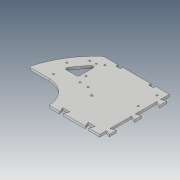
# Autodesk Inventor part: FR_bottomPlate
Saved by Autodesk Inventor 2018 (Build 220112000, 112)
## iProperties
Created: 2020-01-08
Part Number: FR_bottomPlate
Material: Generic
Document SubType Name: Modeling
Designer: anirudh
Density: 1 g/cm^3
Appearance: Default
Author: anirudh
Autodesk Inventor part; units mm, degrees
ref_plane "YZ Plane" through (0, 0, 0) normal (1, 0, 0) x (0, 1, 0)
ref_plane "XZ Plane" through (0, 0, 0) normal (0, 1, 0) x (-1, 0, 0)
ref_plane "XY Plane" through (0, 0, 0) normal (0, 0, 1) x (1, 0, 0)
sketch "Sketch1" plane through (0, 0, 0) normal (0, 1, 0) x (-1, 0, 0)
  arc A0 (-134.4042, 152.4) -> (-189.4285, 73.533) centre (0, 0) ccw
  arc A1 (-189.4285, -73.533) -> (-134.4042, -152.4) centre (0, 0) ccw
  arc A2 (-134.4042, 152.4) -> (-189.4285, 73.533) centre (0, 0) ccw
  arc A3 (-189.4285, -73.533) -> (-134.4042, -152.4) centre (0, 0) ccw
  arc A4 (214.8285, 73.533) -> (159.8042, 152.4) centre (25.4, 0) ccw
  arc A5 (159.8042, -152.4) -> (214.8285, -73.533) centre (25.4, 0) ccw
  arc A6 (214.8285, 73.533) -> (159.8042, 152.4) centre (25.4, 0) ccw
  arc A7 (159.8042, -152.4) -> (214.8285, -73.533) centre (25.4, 0) ccw
  arc A8 (-152.4, -50.8) -> (-152.4, 50.8) centre (-152.4, 0) ccw
  arc A9 (177.8, 50.8) -> (177.8, -50.8) centre (177.8, 0) ccw
  line L0 (177.8, 50.8) -> (222.1476, 50.8)
  line L1 (177.8, -50.8) -> (222.1476, -50.8)
  line L2 (-152.4, 50.8) -> (-196.7476, 50.8)
  line L3 (-152.4, -50.8) -> (-196.7476, -50.8)
  arc A10 (-134.4042, 152.4) -> (-196.7476, 50.8) centre (0, 0) ccw
  arc A11 (-196.7476, -50.8) -> (-134.4042, -152.4) centre (0, 0) ccw
  arc A12 (159.8042, -152.4) -> (222.1476, -50.8) centre (25.4, 0) ccw
  arc A13 (222.1476, 50.8) -> (159.8042, 152.4) centre (25.4, 0) ccw
  circle A14 centre (98.425, -65.0875) radius 2.1
  circle A15 centre (98.425, 65.0875) radius 2.1
  circle A16 centre (-73.025, 65.0875) radius 2.1
  circle A17 centre (-73.025, -65.0875) radius 2.1
  line L4 (-20.32, 152.4) -> (-20.32, 147.32)
  line L5 (-20.32, 147.32) -> (-30.48, 147.32)
  line L6 (-30.48, 147.32) -> (-30.48, 152.4)
  line L7 (-92.5481, 152.4) -> (-92.5481, 147.32)
  line L8 (-92.5481, 147.32) -> (-102.7081, 147.32)
  line L9 (-102.7081, 147.32) -> (-102.7081, 152.4)
  line L10 (-102.7081, 152.4) -> (-134.4042, 152.4)
  line L11 (-60.8521, 152.4) -> (-92.5481, 152.4)
  line L12 (-102.7081, 152.4) -> (-134.4042, 152.4)
  line L13 (-134.4042, 152.4) -> (-102.7081, 152.4)
  line L14 (12.7, 152.4) -> (-20.32, 152.4)
  line L15 (-30.48, 152.4) -> (-60.8521, 152.4)
  line L16 (12.7, 152.4) -> (-20.32, 152.4)
  line L17 (-30.48, 152.4) -> (-92.5481, 152.4)
  line L18 (-92.5481, 152.4) -> (-30.48, 152.4)
  line L19 (-20.32, 152.4) -> (12.7, 152.4)
  line L20 (45.72, 152.4) -> (45.72, 147.32)
  line L21 (45.72, 147.32) -> (55.88, 147.32)
  line L22 (55.88, 147.32) -> (55.88, 152.4)
  line L23 (117.9481, 152.4) -> (117.9481, 147.32)
  line L24 (117.9481, 147.32) -> (128.1081, 147.32)
  line L25 (128.1081, 147.32) -> (128.1081, 152.4)
  line L26 (-20.32, -152.4) -> (-20.32, -147.32)
  line L27 (-20.32, -147.32) -> (-30.48, -147.32)
  line L28 (-30.48, -147.32) -> (-30.48, -152.4)
  line L29 (-92.5481, -152.4) -> (-92.5481, -147.32)
  line L30 (-92.5481, -147.32) -> (-102.7081, -147.32)
  line L31 (-102.7081, -147.32) -> (-102.7081, -152.4)
  line L32 (55.88, -147.32) -> (55.88, -152.4)
  line L33 (45.72, -147.32) -> (55.88, -147.32)
  line L34 (45.72, -152.4) -> (45.72, -147.32)
  line L35 (117.9481, -147.32) -> (128.1081, -147.32)
  line L36 (128.1081, -147.32) -> (128.1081, -152.4)
  line L37 (117.9481, -152.4) -> (117.9481, -147.32)
  line L38 (128.1081, 152.4) -> (159.8042, 152.4)
  line L39 (12.7, 152.4) -> (45.72, 152.4)
  line L40 (55.88, 152.4) -> (117.9481, 152.4)
  line L41 (-102.7081, -152.4) -> (-134.4042, -152.4)
  line L42 (12.7, -152.4) -> (-20.32, -152.4)
  line L43 (-30.48, -152.4) -> (-92.5481, -152.4)
  line L44 (12.7, -152.4) -> (45.72, -152.4)
  line L45 (55.88, -152.4) -> (117.9481, -152.4)
  line L46 (128.1081, -152.4) -> (159.8042, -152.4)
  point P0 (-25.4, -152.4)
  point P1 (50.8, 152.4)
  point P2 (50.8, -152.4)
  point P3 (50.8, -152.4)
  dimension "d22" = 101.6
  dimension "d31" = 4.2
  dimension "d32" = 4.2
  dimension "d34" = 4.2
  constraints: 94 end point, 28 point on circle, 18 centre point, 15 collinear, 12 point on line, 7 perpendicular, 4 coincident, 2 tangent, 1 vertical
  measures "d22" diameter of A9
  measures "d31" diameter of A14
  measures "d32" diameter of A15
  measures "d34" diameter of A17
extrude "Extrusion2" add sketch "Sketch1" along normal blind 5.08
sketch "Sketch2" plane through (0, 5.08, 0) normal (0, 1, 0) x (1, 0, 0)
  arc A0 (-177.8, -50.8) -> (-177.8, 50.8) centre (-177.8, 0) ccw projected
  arc A1 (152.4, 50.8) -> (152.4, -50.8) centre (152.4, 0) ccw projected
  line L0 (-177.8, 0) -> (152.4, 0)
  line L1 (-12.7, 0) -> (-12.7, -152.4)
  line L2 (-12.7, 0) -> (-12.7, 152.4)
  line L3 (20.32, 152.4) -> (-45.72, 152.4) projected
  point P0 (0, 0)
  constraints: 6 end point, 2 midpoint, 1 horizontal
sketch "Sketch4" plane through (0, 5.08, 0) normal (0, 1, 0) x (1, 0, 0)
  circle A0 centre (-12.7, 0) radius 300
  point P0 (-177.8, 0)
  point P1 (152.4, 0)
  constraints: 1 centre point
sketch "Sketch5" plane through (0, 5.08, 0) normal (0, 1, 0) x (1, 0, 0)
  line L0 (101.6, 0) -> (80.9498, 0)
  arc A0 (-177.8, -50.8) -> (-177.8, 50.8) centre (-177.8, 0) ccw projected
  line L1 (-106.3498, 0) -> (-106.3498, -74.5998)
  line L2 (30.48, -152.4) -> (92.5481, -152.4) projected
  line L3 (80.9498, -74.5998) -> (-106.3498, -74.5998)
  line L4 (-55.88, 152.4) -> (-117.9481, 152.4) projected
  line L5 (-106.3498, 74.5998) -> (80.9498, 74.5998)
  circle A1 centre (9.525, -102.362) radius 1.75 projected
  line L6 (20.32, 152.4) -> (-45.72, 152.4) projected
  circle A2 centre (-34.925, -140.4366) radius 1.75 projected
  line L7 (-41.3004, -140.4366) -> (-41.3004, -152.4)
  line L8 (-45.72, -152.4) -> (20.32, -152.4) projected
  circle A3 centre (-34.925, -102.362) radius 1.75 projected
  line L9 (-34.925, -89.6366) -> (-41.3004, -89.6366)
  line L10 (-41.3004, -89.6366) -> (15.9004, -89.6366)
  circle A4 centre (-34.925, 102.362) radius 1.75 projected
  line L11 (-34.925, 89.6366) -> (-41.3004, 89.6366)
  line L12 (-41.3004, 89.6366) -> (15.9004, 89.6366)
  line L13 (-41.3004, -152.4) -> (-41.3004, -89.6366)
  line L14 (-41.3004, 89.6366) -> (-41.3004, 152.4)
  line L15 (15.9004, -152.4) -> (15.9004, -89.6366)
  line L16 (15.9004, 89.6366) -> (15.9004, 152.4)
  line L17 (80.9498, -74.5998) -> (80.9498, 74.5998)
  line L18 (80.9498, 0) -> (80.9498, -74.5998)
  line L19 (-106.3498, -74.5998) -> (-106.3498, 74.5998)
  arc A5 (134.4042, -152.4) -> (196.7476, -50.8) centre (0, 0) ccw projected
  line L20 (102.7081, -152.4) -> (134.4042, -152.4) projected
  line L21 (80.9498, -74.5998) -> (80.9498, -68.2498)
  line L22 (84.1248, -68.2498) -> (119.6848, -68.2498)
  line L23 (119.6848, -68.2498) -> (119.6848, -86.0298)
  line L24 (119.6848, -86.0298) -> (84.1248, -86.0298)
  line L25 (84.1248, -86.0298) -> (84.1248, -68.2498)
  line L26 (152.4, 0) -> (-177.8, 0)
  line L27 (-12.7, 0) -> (-12.7, 50.8)
  line L28 (-109.5248, -68.2498) -> (-145.0848, -68.2498)
  line L29 (-145.0848, -68.2498) -> (-145.0848, -86.0298)
  line L30 (-145.0848, -86.0298) -> (-109.5248, -86.0298)
  line L31 (-109.5248, -86.0298) -> (-109.5248, -68.2498)
  line L32 (84.1248, 68.2498) -> (119.6848, 68.2498)
  line L33 (119.6848, 68.2498) -> (119.6848, 86.0298)
  line L34 (119.6848, 86.0298) -> (84.1248, 86.0298)
  line L35 (84.1248, 86.0298) -> (84.1248, 68.2498)
  line L36 (-109.5248, 86.0298) -> (-109.5248, 68.2498)
  line L37 (-145.0848, 86.0298) -> (-109.5248, 86.0298)
  line L38 (-145.0848, 68.2498) -> (-145.0848, 86.0298)
  line L39 (-109.5248, 68.2498) -> (-145.0848, 68.2498)
  line L40 (15.9004, -152.4) -> (15.9004, -133.35)
  line L41 (80.9498, -74.5998) -> (63.1698, -74.5998)
  line L42 (63.1698, -82.1182) -> (63.1698, -133.35)
  line L43 (63.1698, -133.35) -> (15.9004, -133.35)
  line L44 (0, -82.1182) -> (63.1698, -82.1182)
  line L45 (84.1248, -133.35) -> (117.6036, -133.35)
  line L46 (84.1248, -133.35) -> (84.1248, -86.0298)
  line L47 (84.1248, -86.0298) -> (155.6011, -86.0298)
  arc A6 (134.4042, -152.4) -> (196.7476, -50.8) centre (0, 0) ccw projected
  arc A7 (117.6036, -133.35) -> (155.6011, -86.0298) centre (0, 0) ccw
  line L48 (63.1698, 82.1182) -> (63.1698, 133.35)
  line L49 (63.1698, 133.35) -> (15.9004, 133.35)
  line L50 (0, 82.1182) -> (63.1698, 82.1182)
  line L51 (84.1248, 133.35) -> (117.6036, 133.35)
  line L52 (84.1248, 133.35) -> (84.1248, 86.0298)
  line L53 (84.1248, 86.0298) -> (155.6011, 86.0298)
  arc A8 (155.6011, 86.0298) -> (117.6036, 133.35) centre (0, 0) ccw
  line L54 (-88.5698, -82.1182) -> (-88.5698, -133.35)
  line L55 (-88.5698, -133.35) -> (-41.3004, -133.35)
  line L56 (-25.4, -82.1182) -> (-88.5698, -82.1182)
  line L57 (-109.5248, -133.35) -> (-143.0036, -133.35)
  line L58 (-109.5248, -133.35) -> (-109.5248, -86.0298)
  line L59 (-109.5248, -86.0298) -> (-181.0011, -86.0298)
  arc A9 (-181.0011, -86.0298) -> (-143.0036, -133.35) centre (-25.4, 0) ccw
  line L60 (-88.5698, 133.35) -> (-41.3004, 133.35)
  line L61 (-88.5698, 82.1182) -> (-88.5698, 133.35)
  line L62 (-25.4, 82.1182) -> (-88.5698, 82.1182)
  line L63 (-109.5248, 133.35) -> (-143.0036, 133.35)
  line L64 (-109.5248, 133.35) -> (-109.5248, 86.0298)
  line L65 (-109.5248, 86.0298) -> (-181.0011, 86.0298)
  arc A10 (-143.0036, 133.35) -> (-181.0011, 86.0298) centre (-25.4, 0) ccw
  line L66 (-41.3004, -133.35) -> (-88.5698, -133.35)
  line L67 (-88.5698, -133.35) -> (-88.5698, -82.1182)
  line L68 (-88.5698, -82.1182) -> (-25.4, -82.1182)
  line L69 (-25.4, -89.6366) -> (-41.3004, -89.6366)
  line L70 (-41.3004, -89.6366) -> (-41.3004, -133.35)
  line L71 (-25.4, -82.1182) -> (0, -82.1182)
  line L72 (-25.4, -89.6366) -> (0, -89.6366)
  line L73 (0, 82.1182) -> (-25.4, 82.1182)
  line L74 (-25.4, 82.1182) -> (-88.5698, 82.1182)
  line L75 (-88.5698, 82.1182) -> (-88.5698, 133.35)
  line L76 (-88.5698, 133.35) -> (-41.3004, 133.35)
  line L77 (-41.3004, 133.35) -> (-41.3004, 89.6366)
  line L78 (-41.3004, 89.6366) -> (-25.4, 89.6366)
  line L79 (15.9004, -133.35) -> (15.9004, -89.6366)
  line L80 (15.9004, -89.6366) -> (-41.3004, -89.6366)
  line L81 (15.9004, 133.35) -> (63.1698, 133.35)
  line L82 (63.1698, 133.35) -> (63.1698, 82.1182)
  line L83 (63.1698, 82.1182) -> (-88.5698, 82.1182)
  line L84 (-88.5698, 82.1182) -> (-88.5698, 133.35)
  line L85 (-88.5698, 133.35) -> (-41.3004, 133.35)
  line L86 (-41.3004, 133.35) -> (-41.3004, 89.6366)
  line L87 (-41.3004, 89.6366) -> (15.9004, 89.6366)
  line L88 (15.9004, 89.6366) -> (15.9004, 133.35)
  constraints: 168 end point, 35 symmetric about line, 20 perpendicular, 9 point on line, 8 collinear, 8 point on circle, 7 horizontal, 4 centre point, 4 parallel, 1 midpoint, 1 vertical, 3 other
ref_plane "Work Plane1" through (134.4042, 0, 0) normal (0, 0, -1) x (-1, 0, 0)
sketch "Sketch6" plane through (0, 5.08, 0) normal (0, 1, 0) x (1, 0, 0)
  arc A0 (196.7476, 50.8) -> (134.4042, 152.4) centre (0, 0) ccw projected
  arc A1 (152.4, 50.8) -> (152.4, -50.8) centre (152.4, 0) ccw projected
  arc A2 (-177.8, -50.8) -> (-177.8, 50.8) centre (-177.8, 0) ccw projected
  line L0 (-45.72, -152.4) -> (20.32, -152.4) projected
  line L1 (20.32, 152.4) -> (-45.72, 152.4) projected
  circle A3 centre (93.0022, 80.3402) radius 1.75
  circle A4 centre (110.7822, 80.3402) radius 1.75
  line L2 (152.4, 0) -> (-177.8, 0)
  line L3 (-12.7, -152.4) -> (-12.7, 152.4)
  circle A5 centre (93.0022, -80.3402) radius 1.75
  circle A6 centre (110.7822, -80.3402) radius 1.75
  circle A7 centre (-118.4022, 80.3402) radius 1.75
  circle A8 centre (-136.1822, 80.3402) radius 1.75
  circle A9 centre (-118.4022, -80.3402) radius 1.75
  circle A10 centre (-136.1822, -80.3402) radius 1.75
  dimension "d86" = 3.5
  dimension "d87" = 3.5
  constraints: 8 centre point, 6 symmetric about line, 4 end point, 2 midpoint, 1 horizontal, 6 other
  measures "d86" diameter of A3
  measures "d87" diameter of A4
extrude "Extrusion4" cut sketch "Sketch6" against normal blind 25.4
extrude "Extrusion5" cut sketch "Sketch5" against normal blind 25.4 contours L49 L48 L50 L73 L62 L61 L60 L14 L11 L12 L16 | L55 L54 L56 L71 L44 L42 L43 L15 L10 L9 L13 | L24 L47 A7 L45 L46 | L58 L57 A9 L59 L30 | L52 L51 A8 L53 L34 | L37 L65 A10 L63 L64
fillet "Fillet2" radius 3.175 28 edges at (63.1698, 2.54, 133.35) (15.9004, 2.54, 133.35) (63.1698, 2.54, 82.1182) (-41.3004, 2.54, 133.35) (-88.5698, 2.54, 133.35) (-88.5698, 2.54, 82.1182) (63.1698, 2.54, -82.1182) (63.1698, 2.54, -133.35) (15.9004, 2.54, -133.35) (-41.3004, 2.54, -133.35) (-88.5698, 2.54, -82.1182) (-88.5698, 2.54, -133.35) (155.6011, 2.54, 86.0298) (84.1248, 2.54, 133.35) (84.1248, 2.54, 86.0298) (117.6036, 2.54, 133.35) (155.6011, 2.54, -86.0298) (117.6036, 2.54, -133.35) (84.1248, 2.54, -133.35) (84.1248, 2.54, -86.0298) (-109.5248, 2.54, 86.0298) (-109.5248, 2.54, 133.35) (-143.0036, 2.54, 133.35) (-181.0011, 2.54, 86.0298) (-109.5248, 2.54, -86.0298) (-109.5248, 2.54, -133.35) (-143.0036, 2.54, -133.35) (-181.0011, 2.54, -86.0298)
fillet "Fillet3" radius 3.175 4 edges at (196.7476, 2.54, 50.8) (196.7476, 2.54, -50.8) (-222.1476, 2.54, 50.8) (-222.1476, 2.54, -50.8)
sketch "Sketch7" plane through (0, 5.08, 0) normal (0, 1, 0) x (1, 0, 0)
  arc A0 (152.4, 50.8) -> (152.4, -50.8) centre (152.4, 0) ccw projected
  circle A1 centre (152.4, -63.5) radius 1.75
  circle A2 centre (152.4, 63.5) radius 1.75
  arc A3 (-177.8, -50.8) -> (-177.8, 50.8) centre (-177.8, 0) ccw projected
  line L0 (152.4, 0) -> (-177.8, 0)
  circle A4 centre (-177.8, -63.5) radius 1.75
  circle A5 centre (-177.8, 63.5) radius 1.75
  dimension "d101" = 3.5
  dimension "d102" = 3.5
  constraints: 4 centre point, 2 end point, 1 horizontal
  measures "d101" diameter of A1
  measures "d102" diameter of A2
extrude "Extrusion6" cut sketch "Sketch7" against normal blind 25.4
sketch "Sketch8" plane through (0, 5.08, 0) normal (0, 1, 0) x (1, 0, 0)
  line L0 (-159.8042, -152.4) -> (-128.1081, -152.4) projected
  line L1 (-159.8042, -152.4) -> (-128.1081, -152.4)
  line L2 (-128.1081, -147.32) -> (-117.9481, -147.32) projected
  line L3 (-128.1081, -152.4) -> (-128.1081, -147.32)
  line L4 (-117.9481, -147.32) -> (-117.9481, -152.4) projected
  line L5 (-128.1081, -147.32) -> (-117.9481, -147.32)
  line L6 (-117.9481, -152.4) -> (-55.88, -152.4) projected
  line L7 (-117.9481, -147.32) -> (-117.9481, -152.4)
  line L8 (-117.9481, -152.4) -> (-55.88, -152.4)
  line L9 (-55.88, -147.32) -> (-45.72, -147.32) projected
  line L10 (-55.88, -152.4) -> (-55.88, -147.32)
  line L11 (-45.72, -147.32) -> (-45.72, -152.4) projected
  line L12 (-55.88, -147.32) -> (-45.72, -147.32)
  line L13 (-45.72, -152.4) -> (20.32, -152.4) projected
  line L14 (-45.72, -147.32) -> (-45.72, -152.4)
  line L15 (-45.72, -152.4) -> (20.32, -152.4)
  line L16 (20.32, -147.32) -> (30.48, -147.32) projected
  line L17 (20.32, -152.4) -> (20.32, -147.32)
  line L18 (30.48, -147.32) -> (30.48, -152.4) projected
  line L19 (20.32, -147.32) -> (30.48, -147.32)
  line L20 (30.48, -147.32) -> (30.48, -152.4)
  line L21 (30.48, -152.4) -> (92.5481, -152.4) projected
  line L22 (30.48, -152.4) -> (92.5481, -152.4)
  line L23 (92.5481, -147.32) -> (102.7081, -147.32) projected
  line L24 (92.5481, -152.4) -> (92.5481, -147.32)
  line L25 (102.7081, -147.32) -> (102.7081, -152.4) projected
  line L26 (92.5481, -147.32) -> (102.7081, -147.32)
  line L27 (102.7081, -147.32) -> (102.7081, -152.4)
  arc A0 (134.4042, -152.4) -> (195.6623, -54.8317) centre (0, 0) ccw projected
  line L28 (102.7081, -152.4) -> (134.4042, -152.4)
  arc A1 (-221.0623, -54.8317) -> (-159.8042, -152.4) centre (-25.4, 0) ccw projected
  line L29 (134.4042, 152.4) -> (102.7081, 152.4) projected
  line L30 (134.4042, 152.4) -> (102.7081, 152.4)
  line L31 (-128.1081, 152.4) -> (-159.8042, 152.4) projected
  line L32 (-128.1081, 147.32) -> (-128.1081, 152.4) projected
  line L33 (-159.8042, 152.4) -> (-128.1081, 152.4)
  line L34 (-117.9481, 147.32) -> (-128.1081, 147.32) projected
  line L35 (-128.1081, 152.4) -> (-128.1081, 147.32)
  line L36 (-128.1081, 147.32) -> (-117.9481, 147.32)
  line L37 (-55.88, 152.4) -> (-117.9481, 152.4) projected
  line L38 (-117.9481, 147.32) -> (-117.9481, 152.4)
  line L39 (-55.88, 147.32) -> (-55.88, 152.4) projected
  line L40 (-117.9481, 152.4) -> (-55.88, 152.4)
  line L41 (-45.72, 147.32) -> (-55.88, 147.32) projected
  line L42 (-55.88, 152.4) -> (-55.88, 147.32)
  line L43 (-55.88, 147.32) -> (-45.72, 147.32)
  line L44 (20.32, 152.4) -> (-45.72, 152.4) projected
  line L45 (-45.72, 147.32) -> (-45.72, 152.4)
  line L46 (-45.72, 152.4) -> (20.32, 152.4)
  line L47 (30.48, 147.32) -> (20.32, 147.32) projected
  line L48 (20.32, 152.4) -> (20.32, 147.32)
  line L49 (20.32, 147.32) -> (30.48, 147.32)
  line L50 (30.48, 152.4) -> (30.48, 147.32) projected
  line L51 (30.48, 147.32) -> (30.48, 152.4)
  line L52 (92.5481, 147.32) -> (92.5481, 152.4) projected
  line L53 (30.48, 152.4) -> (92.5481, 152.4)
  line L54 (92.5481, 152.4) -> (92.5481, 147.32)
  line L55 (102.7081, 152.4) -> (102.7081, 147.32) projected
  line L56 (92.5481, 147.32) -> (102.7081, 147.32)
  line L57 (102.7081, 147.32) -> (102.7081, 152.4)
  arc A2 (-177.8, -50.8) -> (-177.8, 50.8) centre (-177.8, 0) ccw projected
  arc A3 (-177.8, -50.8) -> (-177.8, 50.8) centre (-177.8, 0) ccw
  arc A4 (152.4, 50.8) -> (152.4, -50.8) centre (152.4, 0) ccw projected
  arc A5 (152.4, 50.8) -> (152.4, -50.8) centre (152.4, 0) ccw
  line L58 (152.4, -50.8) -> (196.7476, -50.8)
  line L59 (152.4, 50.8) -> (196.7476, 50.8)
  line L60 (-177.8, -50.8) -> (-218.005, -50.8) projected
  line L61 (-177.8, -50.8) -> (-222.1476, -50.8)
  line L62 (-218.005, 50.8) -> (-177.8, 50.8) projected
  line L63 (-177.8, 50.8) -> (-222.1476, 50.8)
  arc A6 (-159.8042, 152.4) -> (-222.1476, 50.8) centre (-25.4, 0) ccw
  arc A7 (-222.1476, -50.8) -> (-159.8042, -152.4) centre (-25.4, 0) ccw
  arc A8 (134.4042, -152.4) -> (196.7476, -50.8) centre (0, 0) ccw
  arc A9 (196.7476, 50.8) -> (134.4042, 152.4) centre (0, 0) ccw
  line L64 (-177.8, 0) -> (152.4, 0)
  line L65 (-12.7, -80.645) -> (-93.345, -80.645)
  line L66 (-93.345, -80.645) -> (67.945, -80.645)
  line L67 (67.945, -80.645) -> (67.945, 80.645)
  line L68 (67.945, 80.645) -> (-93.345, 80.645)
  line L69 (-93.345, 80.645) -> (-93.345, -80.645)
  circle A10 centre (-177.8, -63.5) radius 1.75 projected
  circle A11 centre (-177.8, -63.5) radius 1.75
  circle A12 centre (-177.8, 63.5) radius 1.75 projected
  circle A13 centre (-177.8, 63.5) radius 1.75
  circle A14 centre (-136.1822, -80.3402) radius 1.75 projected
  circle A15 centre (-136.1822, -80.3402) radius 1.75
  circle A16 centre (-118.4022, -80.3402) radius 1.75 projected
  circle A17 centre (-118.4022, -80.3402) radius 1.75
  circle A18 centre (-136.1822, 80.3402) radius 1.75 projected
  circle A19 centre (-136.1822, 80.3402) radius 1.75
  circle A20 centre (-118.4022, 80.3402) radius 1.75 projected
  circle A21 centre (-118.4022, 80.3402) radius 1.75
  circle A22 centre (93.0022, -80.3402) radius 1.75 projected
  circle A23 centre (93.0022, -80.3402) radius 1.75
  circle A24 centre (110.7822, -80.3402) radius 1.75 projected
  circle A25 centre (110.7822, -80.3402) radius 1.75
  circle A26 centre (152.4, -63.5) radius 1.75 projected
  circle A27 centre (152.4, -63.5) radius 1.75
  circle A28 centre (152.4, 63.5) radius 1.75 projected
  circle A29 centre (152.4, 63.5) radius 1.75
  circle A30 centre (93.0022, 80.3402) radius 1.75 projected
  circle A31 centre (93.0022, 80.3402) radius 1.75
  circle A32 centre (110.7822, 80.3402) radius 1.75 projected
  circle A33 centre (110.7822, 80.3402) radius 1.75
  dimension "d106" = 80.645
  dimension "d107" = 161.29
  constraints: 89 end point, 30 perpendicular, 18 centre point, 16 coincident, 14 point on circle, 7 horizontal, 4 collinear, 4 point on line, 2 parallel, 2 tangent
  measures "d106" distance of L65.start L65.end
  measures "d107" distance of L68.end L67.end
sketch "Sketch10" plane through (0, 5.08, 0) normal (0, 1, 0) x (1, 0, 0)
  line L0 (-177.8, -50.8) -> (-218.005, -50.8) projected
  circle A0 centre (-177.8, -63.5) radius 1.75 projected
  arc A1 (-221.0623, -54.8317) -> (-159.8042, -152.4) centre (-25.4, 0) ccw projected
  circle A2 centre (-209.7483, -57.15) radius 1.75
  circle A3 centre (-188.4494, -57.15) radius 1.75
  line L1 (-218.005, 50.8) -> (-177.8, 50.8) projected
  arc A4 (-177.8, -50.8) -> (-177.8, 50.8) centre (-177.8, 0) ccw projected
  circle A5 centre (-177.8, 63.5) radius 1.75 projected
  arc A6 (-159.8042, 152.4) -> (-221.0623, 54.8317) centre (-25.4, 0) ccw projected
  circle A7 centre (-209.7483, 57.15) radius 1.75
  circle A8 centre (-188.4494, 57.15) radius 1.75
  point P0 (0, 0)
  dimension "d109" = 3.5
  dimension "d110" = 3.5
  dimension "d111" = 3.5
  dimension "d112" = 3.5
  constraints: 4 centre point
  measures "d109" diameter of A2
  measures "d110" diameter of A3
  measures "d111" diameter of A7
  measures "d112" diameter of A8
extrude "Extrusion7" cut sketch "Sketch10" against normal blind 25.4 contours A2 | A3 | A7 | A8
sketch "Sketch12" plane through (0, 5.08, 0) normal (0, 1, 0) x (1, 0, 0)
  arc A0 (-177.8, -50.8) -> (-177.8, 50.8) centre (-177.8, 0) ccw projected
  line L0 (-127, 0) -> (-106.6679, 0)
  circle A1 centre (-116.8339, 0) radius 1.75
  circle A2 centre (-116.8339, 57.15) radius 1.75
  circle A3 centre (-116.8339, -57.15) radius 1.75
  arc A4 (152.4, 50.8) -> (152.4, -50.8) centre (152.4, 0) ccw projected
  circle A5 centre (91.44, 57.15) radius 1.75
  circle A6 centre (91.44, 0) radius 1.75
  circle A7 centre (91.44, -57.15) radius 1.75
  point P0 (0, 0)
  dimension "d120" = 3.5
  dimension "d123" = 3.5
  dimension "d124" = 3.5
  dimension "d128" = 3.5
  dimension "d129" = 3.5
  dimension "d130" = 3.5
  constraints: 6 centre point, 2 end point, 1 horizontal, 1 point on circle
  measures "d120" diameter of A1
  measures "d123" diameter of A2
  measures "d124" diameter of A3
  measures "d128" diameter of A5
  measures "d129" diameter of A6
  measures "d130" diameter of A7
extrude "Extrusion8" cut sketch "Sketch12" against normal blind 25.4
ref_plane "Work Plane2" through (-99.0473, 5.08, 89.2048) normal (-1, 0, 0) x (0, 0, 1)
sketch "Sketch17" plane through (0, 5.08, 0) normal (0, 1, 0) x (1, 0, 0)
  line L0 (-41.3004, 89.6366) -> (15.9004, 89.6366) projected
  line L1 (15.9004, 89.6366) -> (-41.3004, 89.6366)
  line L2 (-41.3004, 89.6366) -> (-41.3004, 76.7454)
  line L3 (-41.3004, 76.7454) -> (15.9004, 76.7454)
  line L4 (15.9004, 76.7454) -> (15.9004, 89.6366)
  line L5 (15.9004, -89.6366) -> (-41.3004, -89.6366) projected
  line L6 (15.9004, -89.6366) -> (-41.3004, -89.6366)
  line L7 (-41.3004, -89.6366) -> (-41.3004, -75.6628)
  line L8 (-41.3004, -75.6628) -> (15.9004, -75.6628)
  line L9 (15.9004, -75.6628) -> (15.9004, -89.6366)
  point P0 (0, 0)
  constraints: 16 end point, 4 parallel, 2 horizontal, 2 perpendicular, 1 point on line
extrude "Extrusion16" add sketch "Sketch17" against normal blind 5.08
fillet "Fillet7" radius 3.175 4 edges at (-41.3004, 2.54, -82.1182) (15.9004, 2.54, -82.1182) (-41.3004, 2.54, 82.1182) (15.9004, 2.54, 82.1182)
sketch "Sketch19" plane through (0, 5.08, 0) normal (0, 1, 0) x (1, 0, 0)
  circle A0 centre (-64.9351, 89.7382) radius 1.75
  line L0 (-44.4754, -94.8182) -> (-85.3948, -94.8182)
  circle A1 centre (-64.9351, -88.4682) radius 1.75
  point P0 (0, 0)
  point P1 (-85.3948, 94.8182)
  point P2 (-44.4754, 94.8182)
  dimension "d188" = 3.5
  dimension "d190" = 3.5
  constraints: 2 centre point, 2 end point, 1 horizontal
  measures "d188" diameter of A0
  measures "d190" diameter of A1
extrude "Extrusion18" cut sketch "Sketch19" against normal blind 20.32
sketch "Sketch20" plane through (0, 5.08, 0) normal (0, 1, 0) x (1, 0, 0)
  line L0 (50.4698, 82.1182) -> (63.1698, 82.1182)
  line L1 (59.9948, -133.35) -> (19.0754, -133.35) projected
  line L2 (-85.3948, -133.35) -> (-44.4754, -133.35) projected
  line L3 (-88.5698, -85.2932) -> (-88.5698, -130.175) projected
  line L4 (-75.8698, -82.1182) -> (-88.5698, -82.1182)
  line L5 (-88.5698, -82.1182) -> (-88.5698, -94.8182)
  line L6 (-88.5698, -94.8182) -> (-75.8698, -94.8182)
  line L7 (-75.8698, -94.8182) -> (-75.8698, -82.1182)
  line L8 (63.1698, -82.1182) -> (50.4698, -82.1182)
  line L9 (50.4698, -82.1182) -> (50.4698, -94.8182)
  line L10 (50.4698, -94.8182) -> (63.1698, -94.8182)
  line L11 (63.1698, -94.8182) -> (63.1698, -82.1182)
  line L12 (50.4698, 82.1182) -> (50.4698, 94.8182)
  line L13 (50.4698, 94.8182) -> (63.1698, 94.8182)
  line L14 (63.1698, 94.8182) -> (63.1698, 82.1182)
  line L15 (-149.392, 86.0298) -> (-149.392, 146.3548)
  line L16 (-149.392, 146.3548) -> (-19.2424, 146.3548)
  line L17 (-19.2424, 146.3548) -> (-19.2424, 86.0298)
  line L18 (-19.2424, 86.0298) -> (-149.392, 86.0298)
  line L19 (-112.6998, 133.35) -> (-141.7974, 133.35) projected
  circle A0 centre (56.8198, 88.4682) radius 1.75
  circle A1 centre (56.8198, -88.4682) radius 1.75
  circle A2 centre (-82.2198, -88.4682) radius 1.75
  line L20 (-175.5213, 86.0298) -> (-112.6998, 86.0298) projected
  line L21 (-3.175, 82.1182) -> (-15.875, 82.1182)
  line L22 (-15.875, 82.1182) -> (-15.875, 94.8182)
  line L23 (-15.875, 94.8182) -> (-3.175, 94.8182)
  line L24 (-3.175, 94.8182) -> (-3.175, 82.1182)
  line L25 (15.9004, 85.2932) -> (15.9004, 130.175) projected
  line L26 (-41.3004, 130.175) -> (-41.3004, 85.2932) projected
  circle A3 centre (-9.525, 88.4682) radius 1.75
  line L27 (-149.392, 141.2389) -> (-149.392, 86.0298)
  line L28 (63.1698, 85.2932) -> (63.1698, 130.175) projected
  line L29 (63.1698, -130.175) -> (63.1698, -85.2932) projected
  circle A4 centre (-27.1672, 136.8298) radius 1.75
  circle A5 centre (-27.1672, 95.5548) radius 1.75
  circle A6 centre (-141.4672, 136.8298) radius 1.75
  circle A7 centre (-141.4672, 95.5548) radius 1.75
  point P0 (0, 0)
  point P1 (-84.3172, 103.1875)
  dimension "d220" = 3.5
  dimension "d221" = 3.5
  dimension "d222" = 3.5
  dimension "d223" = 3.5
  constraints: 40 end point, 8 centre point, 8 parallel, 4 perpendicular, 3 horizontal, 1 point on line, 1 vertical, 4 other
  measures "d220" diameter of A4
  measures "d221" diameter of A5
  measures "d222" diameter of A6
  measures "d223" diameter of A7
sketch "Sketch21" plane through (0, 5.08, 0) normal (0, 1, 0) x (1, 0, 0)
  line L0 (-35.3171, 137.3092) -> (-92.9346, 137.3092)
  line L1 (-92.9346, 137.3092) -> (-92.9346, 73.4211)
  line L2 (-92.9346, 73.4211) -> (-35.3171, 73.4211)
  line L3 (-35.3171, 73.4211) -> (-35.3171, 137.3092)
  point P0 (0, 0)
  constraints: 8 end point, 2 parallel, 1 horizontal, 1 perpendicular
extrude "Extrusion19" add sketch "Sketch21" against normal blind 5.08
sketch "Sketch22" plane through (0, 5.08, 0) normal (0, 1, 0) x (1, 0, 0)
  line L0 (-149.3847, 86.0298) -> (-104.6469, 86.0298)
  line L1 (-104.6469, 86.0298) -> (-104.6469, 140.3034)
  line L2 (-104.6469, 140.3034) -> (-149.3847, 140.3034)
  line L3 (-149.3847, 140.3034) -> (-149.3847, 86.0298)
  point P0 (0, 0)
  point P1 (-175.5213, 86.0298)
  constraints: 8 end point, 2 parallel, 1 horizontal, 1 perpendicular
extrude "Extrusion20" add sketch "Sketch22" against normal blind 5.08
fillet "Fillet9" radius 3.175 2 edges at (-149.3847, 2.54, -127.4388) (-149.3847, 2.54, -86.0298)
sketch "Sketch23" plane through (0, 5.08, 0) normal (0, 1, 0) x (1, 0, 0)
  line L0 (63.1698, 82.1182) -> (50.4698, 82.1182)
  line L1 (50.4698, 82.1182) -> (50.4698, 94.8182)
  line L2 (50.4698, 94.8182) -> (63.1698, 94.8182)
  line L3 (63.1698, 94.8182) -> (63.1698, 82.1182)
  line L4 (63.1698, -82.1182) -> (50.4698, -82.1182)
  line L5 (50.4698, -82.1182) -> (50.4698, -94.8182)
  line L6 (50.4698, -94.8182) -> (63.1698, -94.8182)
  line L7 (63.1698, -94.8182) -> (63.1698, -82.1182)
  line L8 (-88.5698, -82.1182) -> (-75.8698, -82.1182)
  line L9 (-75.8698, -82.1182) -> (-75.8698, -94.8182)
  line L10 (-75.8698, -94.8182) -> (-88.5698, -94.8182)
  line L11 (-88.5698, -94.8182) -> (-88.5698, -82.1182)
  point P0 (0, 0)
  dimension "d211" = 12.7
  dimension "d212" = 12.7
  dimension "d213" = 12.7
  dimension "d214" = 12.7
  dimension "d215" = 12.7
  dimension "d216" = 12.7
  constraints: 24 end point, 6 parallel, 3 horizontal, 3 perpendicular, 2 point on line
  measures "d211" distance of L1.end L2.end
  measures "d212" distance of L0.end L1.end
  measures "d213" distance of L6.end L5.end
  measures "d214" distance of L5.end L4.end
  measures "d215" distance of L9.end L10.end
  measures "d216" distance of L8.end L9.end
extrude "Extrusion21" add sketch "Sketch23" against normal blind 5.08
fillet "Fillet10" radius 3.175 9 edges at (63.1698, 2.54, -94.8182) (50.4698, 2.54, -94.8182) (50.4698, 2.54, -82.1182) (50.4698, 2.54, 82.1182) (50.4698, 2.54, 94.8182) (63.1698, 2.54, 94.8182) (-75.8698, 2.54, 82.1182) (-75.8698, 2.54, 94.8182) (-88.5698, 2.54, 94.8182)
extrude "Extrusion22" cut sketch "Sketch20" against normal blind 10.16 contours A0 | A1 | A2 | A3 | A4 | A5 | A6 | A7
sketch "Sketch24" plane through (0, 5.08, 0) normal (0, 1, 0) x (1, 0, 0)
  line L0 (-149.3847, 119.6842) -> (-149.3847, 89.2048) projected
  line L1 (-175.5213, -86.0298) -> (-112.6998, -86.0298) projected
  line L2 (-149.3847, -86.0298) -> (-102.6114, -86.0298)
  line L3 (-102.6114, -86.0298) -> (-102.6114, -137.6759)
  line L4 (-102.6114, -137.6759) -> (-149.3847, -137.6759)
  line L5 (-149.3847, -137.6759) -> (-149.3847, -86.0298)
  point P0 (0, 0)
  constraints: 8 end point, 2 parallel, 1 horizontal, 1 perpendicular, 1 point on line
extrude "Extrusion23" add sketch "Sketch24" against normal blind 5.08
fillet "Fillet11" radius 3.175 2 edges at (-149.3847, 2.54, 127.4388) (-149.3847, 2.54, 86.0298)
sketch "Sketch25" plane through (0, 5.08, 0) normal (0, 1, 0) x (1, 0, 0)
  line L0 (-159.8042, 152.4) -> (-154.8717, 121.8603)
  arc A0 (-154.8717, 121.8603) -> (-178.2507, 90.8267) centre (-25.4, 0) ccw projected
  line L1 (-178.2507, 90.8267) -> (-209.614, 85.7638)
  arc A1 (-154.8717, 121.8603) -> (-178.2507, 90.8267) centre (-25.4, 0) ccw
  arc A2 (-159.8042, 152.4) -> (-209.614, 85.7638) centre (-25.4, 0) ccw
  circle A3 centre (-166.4316, 128.5066) radius 1.75
  circle A4 centre (-187.8284, 100.1043) radius 1.75
  arc A5 (152.4, 50.8) -> (152.4, -50.8) centre (152.4, 0) ccw projected
  line L2 (152.4, 0) -> (-177.8, 0)
  line L3 (134.4042, 152.4) -> (129.4717, 121.8603)
  arc A6 (152.8507, 90.8267) -> (129.4717, 121.8603) centre (0, 0) ccw
  line L4 (152.8507, 90.8267) -> (184.214, 85.7638)
  arc A7 (152.8507, 90.8267) -> (129.4717, 121.8603) centre (0, 0) ccw
  arc A8 (184.214, 85.7638) -> (134.4042, 152.4) centre (0, 0) ccw
  circle A9 centre (141.0316, 128.5066) radius 1.75
  circle A10 centre (162.4284, 100.1043) radius 1.75
  line L5 (-159.8042, -152.4) -> (-154.8717, -121.8603)
  arc A11 (-178.2507, -90.8267) -> (-154.8717, -121.8603) centre (-25.4, 0) ccw
  line L6 (-178.2507, -90.8267) -> (-209.614, -85.7638)
  arc A12 (-178.2507, -90.8267) -> (-154.8717, -121.8603) centre (-25.4, 0) ccw
  arc A13 (-209.614, -85.7638) -> (-159.8042, -152.4) centre (-25.4, 0) ccw
  circle A14 centre (-166.4316, -128.5066) radius 1.75
  circle A15 centre (-187.8284, -100.1043) radius 1.75
  line L7 (134.4042, -152.4) -> (129.4717, -121.8603)
  arc A16 (129.4717, -121.8603) -> (152.8507, -90.8267) centre (0, 0) ccw
  arc A17 (129.4717, -121.8603) -> (152.8507, -90.8267) centre (0, 0) ccw
  circle A18 centre (141.0316, -128.5066) radius 1.75
  arc A19 (134.4042, -152.4) -> (184.214, -85.7638) centre (0, 0) ccw
  line L8 (152.8507, -90.8267) -> (184.214, -85.7638)
  circle A20 centre (162.4284, -100.1043) radius 1.75
  point P0 (-175.5213, 86.0298)
  constraints: 22 point on circle, 19 centre point, 18 end point, 12 symmetric about line, 9 coincident, 1 horizontal, 10 other
extrude "Extrusion24" cut sketch "Sketch25" against normal blind 25.4 contours A3 | A4 | A9 | A10 | A14 | A15 | A18 | A20
sketch "Sketch26" plane through (0, 5.08, 0) normal (0, 1, 0) x (1, 0, 0)
  line L0 (-149.3847, 119.6842) -> (-149.3847, 89.2048) projected
  line L1 (-117.9481, -152.4) -> (-55.88, -152.4) projected
  circle A0 centre (-92.5739, -114.0841) radius 1.75
  circle A1 centre (-117.0886, -114.0841) radius 1.75
  point P0 (0, 0)
  constraints: 2 centre point
extrude "Extrusion25" cut sketch "Sketch26" against normal blind 25.4
sketch "Sketch27" plane through (0, 5.08, 0) normal (0, 1, 0) x (1, 0, 0)
  circle A0 centre (128.2294, 130.175) radius 1.75
  circle A1 centre (118.5546, 137.541) radius 1.75
  circle A2 centre (128.2294, -130.175) radius 1.75
  circle A3 centre (118.5546, -137.541) radius 1.75
  circle A4 centre (-153.6294, 130.175) radius 1.75
  circle A5 centre (-153.6294, -130.175) radius 1.75
  circle A6 centre (-143.9546, -137.541) radius 1.75
  arc A7 (152.4, 50.8) -> (152.4, -50.8) centre (152.4, 0) ccw projected
  line L0 (-177.8, 0) -> (152.4, 0)
  point P0 (0, 0)
  point P1 (-25.4, 0)
  point P2 (102.7081, 152.4)
  point P3 (118.5137, 132.5418)
  point P4 (116.3974, 130.175)
  point P5 (118.5137, -132.5418)
  point P6 (116.3974, -130.175)
  point P7 (-143.9137, -132.5418)
  constraints: 7 centre point, 2 end point, 1 horizontal
extrude "Extrusion26" cut sketch "Sketch27" against normal blind 25.4
sketch "Sketch29" plane through (0, 5.08, 0) normal (0, 1, 0) x (1, 0, 0)
  circle A0 centre (-116.8339, -57.15) radius 1.75 projected
  circle A1 centre (-116.8339, -57.15) radius 1.75
  circle A2 centre (-116.8339, 0) radius 1.75 projected
  circle A3 centre (-116.8339, 0) radius 1.75
  circle A4 centre (-116.8339, 57.15) radius 1.75 projected
  circle A5 centre (-116.8339, 57.15) radius 1.75
  circle A6 centre (91.44, -57.15) radius 1.75 projected
  circle A7 centre (91.44, -57.15) radius 1.75
  circle A8 centre (91.44, 0) radius 1.75 projected
  circle A9 centre (91.44, 0) radius 1.75
  circle A10 centre (91.44, 57.15) radius 1.75 projected
  circle A11 centre (91.44, 57.15) radius 1.75
  point P0 (0, 0)
  constraints: 6 centre point, 6 coincident
extrude "Extrusion27" add sketch "Sketch29" against normal blind 5.08
sketch "Sketch30" plane through (0, 5.08, 0) normal (0, 1, 0) x (1, 0, 0)
  circle A0 centre (-209.7483, -57.15) radius 1.75 projected
  circle A1 centre (-209.7483, -57.15) radius 1.75
  circle A2 centre (-188.4494, -57.15) radius 1.75 projected
  circle A3 centre (-188.4494, -57.15) radius 1.75
  circle A4 centre (-188.4494, 57.15) radius 1.75 projected
  circle A5 centre (-188.4494, 57.15) radius 1.75
  circle A6 centre (-209.7483, 57.15) radius 1.75 projected
  circle A7 centre (-209.7483, 57.15) radius 1.75
  point P0 (0, 0)
  constraints: 4 centre point, 4 coincident
extrude "Extrusion28" add sketch "Sketch30" against normal blind 5.08
sketch "Sketch31" plane through (0, 5.08, 0) normal (0, 1, 0) x (1, 0, 0)
  circle A0 centre (-180.7464, -63.5) radius 1.75
  circle A1 centre (-180.7464, 63.5) radius 1.75
  circle A2 centre (155.3464, -63.5) radius 1.75
  circle A3 centre (155.3464, 63.5) radius 1.75
  point P0 (0, 0)
  point P1 (-177.8, -63.5)
  point P2 (152.4, 63.5)
  dimension "d258" = 3.5
  dimension "d259" = 3.5
  dimension "d260" = 3.5
  constraints: 4 centre point
  measures "d258" diameter of A0
  measures "d259" diameter of A1
  measures "d260" diameter of A2
sketch "Sketch32" plane through (0, 5.08, 0) normal (0, 1, 0) x (1, 0, 0)
  circle A0 centre (-177.8, -63.5) radius 1.75 projected
  circle A1 centre (-177.8, -63.5) radius 1.75
  circle A2 centre (-177.8, 63.5) radius 1.75 projected
  circle A3 centre (-177.8, 63.5) radius 1.75
  circle A4 centre (152.4, -63.5) radius 1.75 projected
  circle A5 centre (152.4, -63.5) radius 1.75
  circle A6 centre (152.4, 63.5) radius 1.75 projected
  circle A7 centre (152.4, 63.5) radius 1.75
  point P0 (0, 0)
  constraints: 4 centre point, 4 coincident
extrude "Extrusion29" add sketch "Sketch32" against normal blind 5.08
extrude "Extrusion30" cut sketch "Sketch31" against normal blind 5.08
sketch "Sketch33" plane through (0, 5.08, 0) normal (0, 1, 0) x (1, 0, 0)
  circle A0 centre (-136.1822, -80.3402) radius 1.75 projected
  circle A1 centre (-118.4022, -80.3402) radius 1.75 projected
  circle A2 centre (-136.1822, 80.3402) radius 1.75 projected
  circle A3 centre (-118.4022, 80.3402) radius 1.75 projected
  circle A4 centre (93.0022, -80.3402) radius 1.75 projected
  circle A5 centre (110.7822, -80.3402) radius 1.75 projected
  circle A6 centre (110.7822, 80.3402) radius 1.75 projected
  circle A7 centre (93.0022, 80.3402) radius 1.75 projected
  circle A8 centre (-136.1822, -77.1398) radius 1.75
  circle A9 centre (-118.4022, -77.1398) radius 1.75
  circle A10 centre (-136.1822, 77.1398) radius 1.75
  circle A11 centre (-118.4022, 77.1398) radius 1.75
  circle A12 centre (93.0022, 77.1398) radius 1.75
  circle A13 centre (110.7822, 77.1398) radius 1.75
  circle A14 centre (93.0022, -77.1398) radius 1.75
  circle A15 centre (110.7822, -77.1398) radius 1.75
  point P0 (0, 0)
  dimension "d272" = 3.5
  dimension "d273" = 3.5
  dimension "d274" = 3.5
  dimension "d275" = 3.5
  dimension "d276" = 3.5
  dimension "d277" = 3.5
  dimension "d278" = 3.5
  dimension "d279" = 3.5
  constraints: 8 centre point
  measures "d272" diameter of A8
  measures "d273" diameter of A9
  measures "d274" diameter of A10
  measures "d275" diameter of A11
  measures "d276" diameter of A12
  measures "d277" diameter of A13
  measures "d278" diameter of A14
  measures "d279" diameter of A15
sketch "Sketch34" plane through (0, 5.08, 0) normal (0, 1, 0) x (1, 0, 0)
  circle A0 centre (-136.1822, -80.3402) radius 1.75 projected
  circle A1 centre (-136.1822, -80.3402) radius 1.75
  circle A2 centre (-118.4022, -80.3402) radius 1.75 projected
  circle A3 centre (-118.4022, -80.3402) radius 1.75
  circle A4 centre (-136.1822, 80.3402) radius 1.75 projected
  circle A5 centre (-136.1822, 80.3402) radius 1.75
  circle A6 centre (-118.4022, 80.3402) radius 1.75 projected
  circle A7 centre (-118.4022, 80.3402) radius 1.75
  circle A8 centre (93.0022, -80.3402) radius 1.75 projected
  circle A9 centre (93.0022, -80.3402) radius 1.75
  circle A10 centre (110.7822, -80.3402) radius 1.75 projected
  circle A11 centre (110.7822, -80.3402) radius 1.75
  circle A12 centre (110.7822, 80.3402) radius 1.75 projected
  circle A13 centre (110.7822, 80.3402) radius 1.75
  circle A14 centre (93.0022, 80.3402) radius 1.75 projected
  circle A15 centre (93.0022, 80.3402) radius 1.75
  point P0 (0, 0)
  constraints: 8 centre point, 8 coincident
extrude "Extrusion31" add sketch "Sketch34" against normal blind 5.08
extrude "Extrusion32" cut sketch "Sketch33" against normal blind 5.08 contours A8 A0 | A0 A8 | A9 A1 | A1 A9 | A10 A2 | A2 A10 | A11 A3 | A3 A11 | A14 A4 | A4 A14 | A15 A5 | A5 A15 | A13 A6 | A6 A13 | A12 A7 | A7 A12 picked at (-136.3029, -78.7773) picked at (-136.1595, -76.4651) picked at (-118.5229, -78.7773) picked at (-118.3795, -76.4651) picked at (-136.0615, 78.7773) picked at (-136.1595, 76.4651) picked at (-118.5229, 78.7773) picked at (-118.3795, 76.4651) picked at (92.8815, -78.7773) picked at (93.0249, -76.4651) picked at (110.6615, -78.7773) picked at (110.8049, -76.4651) picked at (110.6615, 78.7773) picked at (110.8049, 76.4651) picked at (92.8815, 78.7773) picked at (93.0249, 76.4651)
sketch "Sketch35" plane through (0, 5.08, 0) normal (0, 1, 0) x (1, 0, 0)
  arc A0 (-177.8, -50.8) -> (-177.8, 50.8) centre (-177.8, 0) ccw projected
  arc A1 (152.4, 50.8) -> (152.4, -50.8) centre (152.4, 0) ccw projected
  circle A2 centre (-9.525, 88.4682) radius 1.75 projected
  line L0 (-15.875, 88.4682) -> (-15.875, 0)
  line L1 (-15.875, 0) -> (-15.875, 185.9932)
  line L2 (-15.875, 0) -> (-249.0638, 0)
  line L3 (212.483, 0) -> (212.483, -191.2674)
  line L4 (212.483, -191.2674) -> (-249.0638, -191.2674)
  line L5 (-249.0638, -191.2674) -> (-249.0638, 0)
  line L6 (-15.875, 185.9932) -> (212.483, 185.9932)
  line L7 (212.483, 185.9932) -> (212.483, 0)
  line L8 (-15.875, 0) -> (-15.875, 185.9932)
  point P0 (0, 0)
  constraints: 18 end point, 2 horizontal, 2 parallel, 1 perpendicular, 1 point on line
extrude "Extrusion33" cut sketch "Sketch35" against normal blind 25.4
sketch "Sketch36" plane through (0, 5.08, 0) normal (0, 1, 0) x (1, 0, 0)
  line L0 (-127, 0) -> (-15.875, 0)
  line L1 (-127, 0) -> (-15.875, 0)
  line L2 (-71.4375, 0) -> (-127, 0)
  line L3 (-71.4375, 0) -> (-15.875, 0)
  line L4 (-95.4088, 0) -> (-91.5988, 10.16)
  line L5 (-99.2188, 0) -> (-95.4088, 0)
  line L6 (-99.2188, 10.16) -> (-91.5988, 10.16)
  line L7 (-99.2188, 10.16) -> (-91.5988, 10.16)
  line L8 (-95.4088, 0) -> (-91.5988, 10.16)
  line L9 (-99.2188, 10.16) -> (-106.8388, 10.16)
  line L10 (-103.0288, 0) -> (-106.8388, 10.16)
  line L11 (-99.2188, 10.16) -> (-106.8388, 10.16)
  line L12 (-103.0288, 0) -> (-106.8388, 10.16)
  line L13 (-99.2188, 0) -> (-103.0288, 0)
  line L14 (-39.8463, 0) -> (-36.0363, 10.16)
  line L15 (-43.6563, 0) -> (-39.8463, 0)
  line L16 (-43.6563, 0) -> (-39.8463, 0)
  line L17 (-43.6563, 10.16) -> (-36.0363, 10.16)
  line L18 (-43.6563, 10.16) -> (-36.0363, 10.16)
  line L19 (-43.6563, 0) -> (-47.4663, 0)
  line L20 (-60.4838, 0) -> (-26.8288, 0)
  line L21 (-60.4838, 0) -> (-26.8288, 0)
  line L22 (-60.4838, 0) -> (-26.8288, 0)
  line L23 (-39.8463, 0) -> (-36.0363, 10.16)
  line L24 (-43.6563, 10.16) -> (-51.2763, 10.16)
  line L25 (-47.4663, 0) -> (-51.2763, 10.16)
  line L26 (-43.6563, 10.16) -> (-51.2763, 10.16)
  line L27 (-47.4663, 0) -> (-51.2763, 10.16)
  line L28 (-43.6563, 0) -> (-47.4663, 0)
  line L29 (-15.875, 0) -> (-15.875, 152.4)
  line L30 (-15.875, 147.32) -> (-15.875, 0)
  line L31 (-15.875, 73.66) -> (-15.875, 147.32)
  line L32 (-15.875, 73.66) -> (-15.875, 0)
  line L33 (-15.875, 110.49) -> (-15.875, 147.32)
  line L34 (-15.875, 110.49) -> (-15.875, 73.66)
  line L35 (-15.875, 73.66) -> (-15.875, 36.83)
  line L36 (-15.875, 36.83) -> (-15.875, 0)
  line L37 (-15.875, 125.095) -> (-5.715, 121.285)
  line L38 (-15.875, 128.905) -> (-15.875, 125.095)
  line L39 (-15.875, 128.905) -> (-15.875, 125.095)
  line L40 (-5.715, 128.905) -> (-5.715, 121.285)
  line L41 (-5.715, 128.905) -> (-5.715, 121.285)
  line L42 (-15.875, 128.905) -> (-15.875, 132.715)
  line L43 (-15.875, 145.7325) -> (-15.875, 112.0775)
  line L44 (-15.875, 145.7325) -> (-15.875, 112.0775)
  line L45 (-15.875, 145.7325) -> (-15.875, 112.0775)
  line L46 (-15.875, 145.7325) -> (-15.875, 112.0775)
  line L47 (-15.875, 125.095) -> (-5.715, 121.285)
  line L48 (-5.715, 128.905) -> (-5.715, 136.525)
  line L49 (-15.875, 132.715) -> (-5.715, 136.525)
  line L50 (-5.715, 128.905) -> (-5.715, 136.525)
  line L51 (-15.875, 132.715) -> (-5.715, 136.525)
  line L52 (-15.875, 128.905) -> (-15.875, 132.715)
  line L53 (-5.715, 73.66) -> (-5.715, 66.04)
  line L54 (-5.715, 73.66) -> (-5.715, 66.04)
  line L55 (-15.875, 69.85) -> (-5.715, 66.04)
  line L56 (-15.875, 73.66) -> (-15.875, 69.85)
  line L57 (-15.875, 69.85) -> (-5.715, 66.04)
  line L58 (-15.875, 73.66) -> (-15.875, 69.85)
  line L59 (-5.715, 73.66) -> (-5.715, 81.28)
  line L60 (-5.715, 73.66) -> (-5.715, 81.28)
  line L61 (-15.875, 73.66) -> (-15.875, 77.47)
  line L62 (-15.875, 73.66) -> (-15.875, 77.47)
  line L63 (-15.875, 77.47) -> (-5.715, 81.28)
  line L64 (-15.875, 90.4875) -> (-15.875, 56.8325)
  line L65 (-15.875, 90.4875) -> (-15.875, 56.8325)
  line L66 (-15.875, 90.4875) -> (-15.875, 56.8325)
  line L67 (-15.875, 90.4875) -> (-15.875, 56.8325)
  line L68 (-15.875, 77.47) -> (-5.715, 81.28)
  line L69 (-5.715, 18.415) -> (-5.715, 10.795)
  line L70 (-5.715, 18.415) -> (-5.715, 10.795)
  line L71 (-15.875, 14.605) -> (-5.715, 10.795)
  line L72 (-15.875, 18.415) -> (-15.875, 14.605)
  line L73 (-15.875, 14.605) -> (-5.715, 10.795)
  line L74 (-15.875, 18.415) -> (-15.875, 14.605)
  line L75 (-5.715, 18.415) -> (-5.715, 26.035)
  line L76 (-5.715, 18.415) -> (-5.715, 26.035)
  line L77 (-15.875, 18.415) -> (-15.875, 22.225)
  line L78 (-15.875, 18.415) -> (-15.875, 22.225)
  line L79 (-15.875, 22.225) -> (-5.715, 26.035)
  line L80 (-15.875, 35.2425) -> (-15.875, 1.5875)
  line L81 (-15.875, 35.2425) -> (-15.875, 1.5875)
  line L82 (-15.875, 35.2425) -> (-15.875, 1.5875)
  line L83 (-15.875, 35.2425) -> (-15.875, 1.5875)
  line L84 (-15.875, 22.225) -> (-5.715, 26.035)
  point P0 (0, 0)
  constraints: 170 end point, 17 point on line, 12 midpoint, 8 collinear
sketch "Sketch37" plane through (0, 5.08, 0) normal (0, 1, 0) x (1, 0, 0)
  line L0 (-127, 0) -> (-15.875, 0)
  line L1 (-127, 0) -> (-15.875, 0)
  line L2 (-71.4375, 0) -> (-127, 0)
  line L3 (-71.4375, 0) -> (-15.875, 0)
  line L4 (-95.4088, 0) -> (-91.5988, 10.16)
  line L5 (-99.2188, 0) -> (-95.4088, 0)
  line L6 (-99.2188, 10.16) -> (-91.5988, 10.16)
  line L7 (-99.2188, 10.16) -> (-91.5988, 10.16)
  line L8 (-95.4088, 0) -> (-91.5988, 10.16)
  line L9 (-99.2188, 10.16) -> (-106.8388, 10.16)
  line L10 (-103.0288, 0) -> (-106.8388, 10.16)
  line L11 (-99.2188, 10.16) -> (-106.8388, 10.16)
  line L12 (-103.0288, 0) -> (-106.8388, 10.16)
  line L13 (-99.2188, 0) -> (-103.0288, 0)
  line L14 (-39.8463, 0) -> (-36.0363, 10.16)
  line L15 (-43.6563, 0) -> (-39.8463, 0)
  line L16 (-43.6563, 0) -> (-39.8463, 0)
  line L17 (-43.6563, 10.16) -> (-36.0363, 10.16)
  line L18 (-43.6563, 10.16) -> (-36.0363, 10.16)
  line L19 (-43.6563, 0) -> (-47.4663, 0)
  line L20 (-60.4838, 0) -> (-26.8288, 0)
  line L21 (-60.4838, 0) -> (-26.8288, 0)
  line L22 (-60.4838, 0) -> (-26.8288, 0)
  line L23 (-39.8463, 0) -> (-36.0363, 10.16)
  line L24 (-43.6563, 10.16) -> (-51.2763, 10.16)
  line L25 (-47.4663, 0) -> (-51.2763, 10.16)
  line L26 (-43.6563, 10.16) -> (-51.2763, 10.16)
  line L27 (-47.4663, 0) -> (-51.2763, 10.16)
  line L28 (-43.6563, 0) -> (-47.4663, 0)
  line L29 (-15.875, 110.49) -> (-15.875, 147.32)
  line L30 (-15.875, 145.7325) -> (-15.875, 112.0775)
  line L31 (-15.875, 145.7325) -> (-15.875, 112.0775)
  line L32 (-15.875, 145.7325) -> (-15.875, 112.0775)
  line L33 (-15.875, 145.7325) -> (-15.875, 112.0775)
  line L34 (-15.875, 128.905) -> (-15.875, 125.095)
  line L35 (-15.875, 128.905) -> (-15.875, 125.095)
  line L36 (-5.715, 128.905) -> (-5.715, 121.285)
  line L37 (-5.715, 128.905) -> (-5.715, 121.285)
  line L38 (-15.875, 125.095) -> (-5.715, 121.285)
  line L39 (-15.875, 125.095) -> (-5.715, 121.285)
  line L40 (-15.875, 18.415) -> (-15.875, 22.225)
  line L41 (-15.875, 18.415) -> (-15.875, 22.225)
  line L42 (-15.875, 22.225) -> (-5.715, 26.035)
  line L43 (-15.875, 22.225) -> (-5.715, 26.035)
  line L44 (-5.715, 18.415) -> (-5.715, 26.035)
  line L45 (-5.715, 18.415) -> (-5.715, 26.035)
  line L46 (-15.875, 0) -> (-15.875, 152.4)
  line L47 (-15.875, 147.32) -> (-15.875, 0)
  line L48 (-15.875, 73.66) -> (-15.875, 147.32)
  line L49 (-15.875, 110.49) -> (-15.875, 73.66)
  line L50 (-15.875, 128.905) -> (-15.875, 132.715)
  line L51 (-15.875, 128.905) -> (-15.875, 132.715)
  line L52 (-5.715, 128.905) -> (-5.715, 136.525)
  line L53 (-5.715, 128.905) -> (-5.715, 136.525)
  line L54 (-15.875, 132.715) -> (-5.715, 136.525)
  line L55 (-15.875, 132.715) -> (-5.715, 136.525)
  line L56 (-15.875, 77.47) -> (-5.715, 81.28)
  line L57 (-15.875, 77.47) -> (-5.715, 81.28)
  line L58 (-5.715, 73.66) -> (-5.715, 81.28)
  line L59 (-5.715, 73.66) -> (-5.715, 81.28)
  line L60 (-15.875, 73.66) -> (-15.875, 77.47)
  line L61 (-15.875, 73.66) -> (-15.875, 77.47)
  line L62 (-15.875, 73.66) -> (-15.875, 69.85)
  line L63 (-15.875, 73.66) -> (-15.875, 69.85)
  line L64 (-15.875, 90.4875) -> (-15.875, 56.8325)
  line L65 (-15.875, 90.4875) -> (-15.875, 56.8325)
  line L66 (-15.875, 90.4875) -> (-15.875, 56.8325)
  line L67 (-15.875, 90.4875) -> (-15.875, 56.8325)
  line L68 (-15.875, 73.66) -> (-15.875, 0)
  line L69 (-15.875, 73.66) -> (-15.875, 36.83)
  line L70 (-5.715, 73.66) -> (-5.715, 66.04)
  line L71 (-5.715, 73.66) -> (-5.715, 66.04)
  line L72 (-15.875, 69.85) -> (-5.715, 66.04)
  line L73 (-15.875, 69.85) -> (-5.715, 66.04)
  line L74 (-5.715, 18.415) -> (-5.715, 10.795)
  line L75 (-5.715, 18.415) -> (-5.715, 10.795)
  line L76 (-15.875, 14.605) -> (-5.715, 10.795)
  line L77 (-15.875, 14.605) -> (-5.715, 10.795)
  line L78 (-15.875, 18.415) -> (-15.875, 14.605)
  line L79 (-15.875, 18.415) -> (-15.875, 14.605)
  line L80 (-15.875, 35.2425) -> (-15.875, 1.5875)
  line L81 (-15.875, 35.2425) -> (-15.875, 1.5875)
  line L82 (-15.875, 36.83) -> (-15.875, 0)
  line L83 (-15.875, 35.2425) -> (-15.875, 1.5875)
  line L84 (-15.875, 35.2425) -> (-15.875, 1.5875)
  point P0 (0, 0)
  point P1 (0, 0)
  constraints: 170 end point, 17 point on line, 12 midpoint, 8 collinear
extrude "Extrusion34" add sketch "Sketch37" against normal blind 5.08 contours L29 L54 L52 L36 L38 | L40 L42 L44 L74 L76 L46 | L46 L56 L58 L70 L72
extrude "Extrusion35" cut sketch "Sketch36" against normal blind 5.08 contours L10 L9 L6 L4 L0 | L25 L24 L17 L14 L0
body "Solid2"
